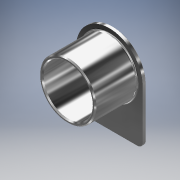
# Autodesk Inventor part: postcap
Saved by Autodesk Inventor 2019 (Build 230136000, 136)
## iProperties
Shininess: 86.0
Length Units: 11272
Angle Units: 11279
Time Units: 11290
Mass Units: 11286
Length Display Precision: 3
Angle Display Precision: 2
Compacted: True
Created: 2001-07-10
Part Number: postcap
Document SubType Name: Modeling
Designer: Autodesk, Inc.
Mass: 3.3995 g
Surface Area: 11.1702 cm^2
Volume: 0.42073 cm^3
Density: 8.08 g/cm^3
Material: Stainless Steel
Appearance: Chrome - Polished
Density: 0.0
Volumn: 0.0
Area: 0.0
PropertySet Name: Model Information
Control State: 0
Master: False
Checked Out: False
Author: Autodesk, Inc.
Autodesk Inventor part; units mm, degrees
ref_plane "Work Plane1" through (0, 0, 0) normal (0, 0, 1) x (1, 0, 0)
ref_plane "Work Plane2" through (-7.9375, -16.2867, 0.7937) normal (0, 0, 1) x (1, 0, 0)
ref_plane "Work Plane3" through (-7.9375, -16.2867, 0.7937) normal (0, 0, 1) x (1, 0, 0)
sketch "Sketch1" plane through (0, 0, 0) normal (0, 0, 1) x (1, 0, 0)
  arc A0 (7.5406, 3.557) -> (-7.5406, 3.557) centre (0, 3.557) ccw projected
  line L0 (7.5406, -7.5872) -> (7.5406, 3.557) projected
  line L1 (-6.3817, -8.7461) -> (6.3818, -8.7461) projected
  arc A1 (6.3818, -8.7461) -> (7.5406, -7.5872) centre (6.3818, -7.5872) ccw projected
  arc A2 (-7.5406, -7.5872) -> (-6.3817, -8.7461) centre (-6.3817, -7.5872) ccw projected
  line L2 (-7.5406, 3.557) -> (-7.5406, -7.5872) projected
extrude "Extrusion2" add sketch "Sketch1" along normal up to surface (0.7937 mm away)
chamfer "Chamfer2" distance 0.127 angle 45 6 edges at (0, -8.7461, 0) (7.2012, -8.4067, 0) (7.5406, -2.0151, 0) (0, 11.0976, 0) (-7.5406, -2.0151, 0) (-7.2012, -8.4067, 0)
sketch "Sketch3" plane through (0, 3.557, 0.7937) normal (0, 0, 1) x (1, 0, 0)
  circle A0 centre (0, 0) radius 6.35
  dimension "d10" = 12.7
  constraints: 1 centre point
  measures "d10" diameter of A0
extrude "Extrusion3" add sketch "Sketch3" along normal blind 9.525
sketch "Sketch4" plane through (0, 3.557, 10.3188) normal (0, 0, 1) x (1, 0, 0)
  circle A0 centre (0, 0) radius 5.5563
  dimension "d13" = 11.1125
  constraints: 1 centre point
  measures "d13" diameter of A0
extrude "Extrusion4" cut sketch "Sketch4" against normal through all
chamfer "Chamfer3" distance 0.254 angle 45 3 edges at (-5.5562, 3.557, 0) (-6.35, 3.557, 10.3187) (-5.5562, 3.557, 10.3188)
fillet "Fillet1" radius 0.381 1 edges at (-6.35, 3.557, 0.7937)
body "Solid1"
